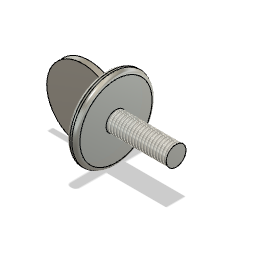
Assembly v1 (Autodesk Fusion 360 archive; units mm, degrees)
design "Pin"
Autodesk Fusion 360 part; units mm, degrees
note: some values were not read from the file. Chosen so that the rebuilt part matches the saved one: a direction; how an offset face is resized.
sketch "Sketch1" plane through (0, 0, 0) normal (1, 0, 0) x (0, 0, -1)
  circle A0 centre (-25, 15) radius 20
  dimension "d1" = 40
  measures "d1" diameter of A0
extrude "Extrude1" add sketch "Sketch1" along normal blind 5
fillet "Fillet1" radius 2 1 edges at (5, 7.7677, 43.6465)
fillet "Fillet2" radius 2 1 edges at (0, 7.7677, 43.6465)
sketch "Sketch2" plane through (5, 0, 0) normal (1, 0, 0) x (0, 0, -1)
  circle A0 centre (-25, 15) radius 18
  circle A1 centre (-25, 15) radius 5
  dimension "d6" = 10
  constraint concentric A0 A1
  measures "d6" diameter of A1
extrude "Extrude2" add sketch "Sketch2" along normal blind 30 contours A1
thread "Thread1" "ISO Metric profile 10.0 M10x1.5 6g" major diameter 9.85 minor diameter 8.141 pitch 1.5 angle 60 resizes the face on face at (25, 14.5022, 20.0248)
sketch "Sketch3" plane through (0, 0, 0) normal (1, 0, 0) x (0, 0, -1)
sketch "Sketch4" plane through (0, 0, 0) normal (-1, 0, 0) x (0, 0, 1)
  circle A0 centre (25, 15) radius 18
sketch "Sketch5" plane through (0, 0, 0) normal (0, 0, 1) x (1, 0, 0)
sketch "Sketch6" plane through (0, 0, 0) normal (0, 0, 1) x (1, 0, 0)
  line L0 (-10, 15) -> (50, 15)
  line L1 (0, 0) -> (0, 29.9666)
  arc A0 (0, 29.9666) -> (0, 0.0334) centre (-10, 15) ccw
  dimension "d9" = 36
  constraint coincident L0.start A0.centre
  constraint coincident L1.start origin
  constraint vertical L1
  constraint coincident L1 A0.end
  measures "d9" diameter of A0
extrude "Extrude3" add sketch "Sketch6" along normal blind 3 from surface at 23.5

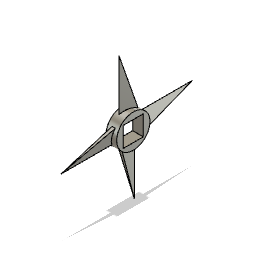
design "Ninja_Star"
Autodesk Fusion 360 part; units mm, degrees
sketch "Sketch1" plane through (0, 0, 0) normal (1, 0, 0) x (0, 0, -1)
  circle A0 centre (0, 0) radius 12.5
  line L0 (7.5, 7.5) -> (-7.5, 7.5)
  line L1 (-7.5, 7.5) -> (-7.5, -7.5)
  line L2 (-7.5, -7.5) -> (7.5, -7.5)
  line L3 (7.5, -7.5) -> (7.5, 7.5)
  line L4 (7.5, 7.5) -> (-7.5, -7.5) construction
  line L5 (-7.5, 7.5) -> (7.5, -7.5) construction
  dimension "d1" = 25
  dimension "d2" = 15
  dimension "d3" = 15
  constraint coincident A0.centre origin
  constraint horizontal L0
  constraint perpendicular L0 L1
  constraint parallel L0 L2
  constraint parallel L1 L3
  constraint coincident L4 A0.centre
  constraint coincident L5 A0.centre
  measures "d1" diameter of A0
  measures "d2" distance of L1.end L2.end
  measures "d3" distance of L0.end L1.end
extrude "Extrude1" add sketch "Sketch1" along normal blind 8
sketch "Sketch2" plane through (0, 0, 0) normal (0, 1, 0) x (1, 0, 0)
sketch "Sketch3" plane through (8, 0, 0) normal (1, 0, 0) x (0, 0, -1)
  line L0 (7.5, 7.5) -> (7.5, -7.5)
  line L1 (7.5, -7.5) -> (-7.5, -7.5)
  line L2 (-7.5, -7.5) -> (-7.5, 7.5)
  line L3 (-7.5, 7.5) -> (7.5, 7.5)
  circle A0 centre (0, 0) radius 12.5
  line L4 (-5.7956, 9.4779) -> (6.4844, 9.4779)
  line L5 (6.4844, 9.4779) -> (-5.7956, 49.4779)
  line L6 (-5.7956, 49.4779) -> (-5.7956, 9.4779)
  dimension "d14" = 40
  constraint perpendicular L0 L4
  constraint perpendicular L4 L6
  measures "d14" distance of L4.start L5.end
extrude "Extrude2" add sketch "Sketch3" along normal blind 2.5 from surface at -5 contours A0 L5 L6
sketch "Sketch4" plane through (0, 0, 0) normal (0, 1, 0) x (1, 0, 0)
  line L0 (2.9867, -5.8624) -> (5.5, -5.8624)
  line L1 (5.5, -5.8624) -> (5.5, 6)
  line L2 (5.5, 6) -> (2.9867, -5.8624)
  constraint horizontal L0
  constraint perpendicular L0 L1
extrude "Extrude3" cut sketch "Sketch4" against normal blind 39 from surface at 50
pattern_circular "C-Pattern1" count 4 over 360 about axis through (1.75, 0, 0) along (1, 0, 0) of "Extrude2", "Extrude3"
sketch "Sketch5" plane through (0, 0, 0) normal (0, 1, 0) x (-1, 0, 0)
sketch "Sketch6" plane through (8, 0, 0) normal (1, 0, 0) x (0, 0, -1)
  line L0 (7.5, 7.5) -> (7.5, -7.5)
  line L1 (7.5, -7.5) -> (-7.5, -7.5)
  line L2 (-7.5, -7.5) -> (-7.5, 7.5)
  line L3 (-7.5, 7.5) -> (7.5, 7.5)
  circle A0 centre (0, 0) radius 12.5
  circle A1 centre (0, 0) radius 12.5
  line L4 (7.5, 7.5) -> (-7.5, 7.5)
  line L5 (-7.5, 7.5) -> (-7.5, -7.5)
  line L6 (-7.5, -7.5) -> (7.5, -7.5)
  line L7 (7.5, -7.5) -> (7.5, 7.5)
  line L8 (7.5, 7.5) -> (-7.5, -7.5) construction
  line L9 (-7.5, 7.5) -> (7.5, -7.5) construction
  constraint coincident A0.centre A1.centre
  constraint horizontal L4
  constraint perpendicular L4 L5
  constraint parallel L4 L6
  constraint parallel L5 L7
  constraint coincident L0.start L3.end
  constraint coincident L8 A0.centre
  constraint coincident L9 A0.centre
extrude "Extrude4" add sketch "Sketch6" against normal blind 8

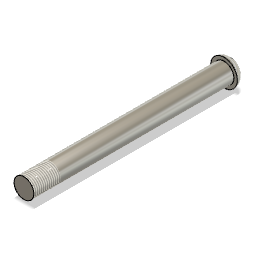
design "HandlePin"
Autodesk Fusion 360 part; units mm, degrees
sketch "Sketch1" plane through (0, 0, 0) normal (0, 0, 1) x (1, 0, 0)
  circle A0 centre (74.2368, 105.6989) radius 7.5
  dimension "d13" = 15
  measures "d13" diameter of A0
extrude "Extrude1" add sketch "Sketch1" along normal blind 150
sketch "Sketch2" plane through (0, 0, 0) normal (0, 0, -1) x (-1, 0, 0)
  circle A0 centre (-74.2368, 105.6989) radius 7.5
  circle A1 centre (-74.2368, 105.6989) radius 10
  dimension "d16" = 20
  constraint horizontal A0.centre A1.centre
  constraint concentric A0 A1
  measures "d16" diameter of A1
extrude "Extrude2" add sketch "Sketch2" along normal blind 6 draft 6 contours A0 | A1
fillet "Fillet1" radius 6 1 edges at (84.148, 109.5431, -6)
sketch "Sketch3" plane through (0, 0, -6) normal (0, 0, -1) x (-1, 0, 0)
  circle A0 centre (-74.2368, 105.6989) radius 4
  line L0 (-75.2368, 112.1989) -> (-73.2368, 112.1989)
  line L1 (-73.2368, 112.1989) -> (-73.2368, 99.1989)
  line L2 (-73.2368, 99.1989) -> (-75.2368, 99.1989)
  line L3 (-75.2368, 99.1989) -> (-75.2368, 112.1989)
  dimension "d20" = 2
  dimension "d21" = 1
  dimension "d22" = 6.5
  constraint horizontal L0
  constraint vertical L1
  constraint horizontal L2
  constraint vertical L3
  measures "d20" distance of L0.start L0.end
  measures "d21" distance of A0.centre L1
  measures "d22" distance of A0.centre L2
extrude "Extrude3" cut sketch "Sketch3" against normal blind 2 contours A0 L1 L3 | A0 L0 L1 L3 | A0 L1 L2 L3
thread "Thread1" "ISO Metric profile 15.0 M15x1.5 6g" major diameter 14.85 minor diameter 13.1369 pitch 1.5 angle 60 resizes the face on face at (81.7275, 105.325, 100)

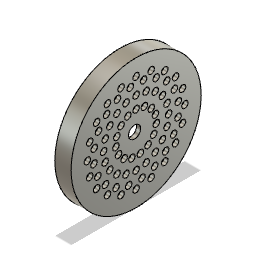
design "SHAPER"
Autodesk Fusion 360 part; units mm, degrees
sketch "Sketch1" plane through (0, 0, 0) normal (1, 0, 0) x (0, 0, -1)
  circle A0 centre (0, 0) radius 80
  circle A1 centre (0, 0) radius 70
  dimension "d1" = 160
  dimension "d2" = 140
  constraint coincident A0.centre A1.centre
  measures "d1" diameter of A0
  measures "d2" diameter of A1
extrude "Extrude1" add sketch "Sketch1" along normal blind 15
thread "Thread1" "ISO Metric profile 140.0 M140x8 6H" major diameter 140.8024 minor diameter 131.8397 pitch 8 angle 60 resizes the face on face at (10, -6.9697, -69.6522)
sketch "Sketch2" plane through (15, 0, 0) normal (1, 0, 0) x (0, 0, -1)
  circle A0 centre (0, 0) radius 65.9198
  circle A1 centre (0, 0) radius 80
  circle A2 centre (0, 0) radius 80
  constraint concentric A0 A2
extrude "Extrude2" add sketch "Sketch2" along normal blind 5 contours A0 | A1 A2
hole "Hole1" at (20, 1.6801, 1.9117) direction (-1, 0, 0) diameter 15 depth 40 tip angle 180
sketch "Sketch3" plane through (20, 0, 0) normal (1, 0, 0) x (0, 0, -1)
  circle A0 centre (-1.9117, 1.6801) radius 7.5
  circle A1 centre (0, 0) radius 80
  point P0 (0, 60)
hole "Hole2" at (20, 60, 0) direction (-1, 0, 0) diameter 8 depth 40 tip angle 180
pattern_circular "C-Pattern1" count 20 over 360 about axis through (1.75, 0, 0) along (1, 0, 0) of "Hole2"
sketch "Sketch4" plane through (20, 0, 0) normal (1, 0, 0) x (0, 0, -1)
  circle A0 centre (18.541, 57.0634) radius 4
  circle A1 centre (35.2671, 48.541) radius 4
  circle A2 centre (48.541, 35.2671) radius 4
  circle A3 centre (57.0634, 18.541) radius 4
  circle A4 centre (60, 0) radius 4
  circle A5 centre (57.0634, -18.541) radius 4
  circle A6 centre (48.541, -35.2671) radius 4
  circle A7 centre (35.2671, -48.541) radius 4
  circle A8 centre (18.541, -57.0634) radius 4
  circle A9 centre (0, -60) radius 4
  circle A10 centre (-18.541, -57.0634) radius 4
  circle A11 centre (-35.2671, -48.541) radius 4
  circle A12 centre (-48.541, -35.2671) radius 4
  circle A13 centre (-57.0634, -18.541) radius 4
  circle A14 centre (-60, 0) radius 4
  circle A15 centre (-57.0634, 18.541) radius 4
  circle A16 centre (-48.541, 35.2671) radius 4
  circle A17 centre (-35.2671, 48.541) radius 4
  circle A18 centre (-18.541, 57.0634) radius 4
  circle A19 centre (0, 60) radius 4
  circle A20 centre (-1.9117, 1.6801) radius 7.5
  circle A21 centre (0, 0) radius 80
  point P0 (-7.2239, 51.8768)
hole "Hole3" at (20, 51.8768, 7.2239) direction (-1, 0, 0) diameter 8 depth 40 tip angle 180
pattern_circular "C-Pattern2" count 20 over 360 about axis through (1.75, 0, 0) along (1, 0, 0) of "Hole3"
sketch "Sketch5" plane through (20, 0, 0) normal (1, 0, 0) x (0, 0, -1)
  circle A0 centre (9.1605, 51.5701) radius 4
  circle A1 centre (24.6482, 46.2153) radius 4
  circle A2 centre (37.7231, 36.3367) radius 4
  circle A3 centre (47.1055, 22.9012) radius 4
  circle A4 centre (51.8768, 7.2239) radius 4
  circle A5 centre (51.5701, -9.1605) radius 4
  circle A6 centre (46.2153, -24.6482) radius 4
  circle A7 centre (36.3367, -37.7231) radius 4
  circle A8 centre (22.9012, -47.1055) radius 4
  circle A9 centre (7.2239, -51.8768) radius 4
  circle A10 centre (-9.1605, -51.5701) radius 4
  circle A11 centre (-24.6482, -46.2153) radius 4
  circle A12 centre (-37.7231, -36.3367) radius 4
  circle A13 centre (-47.1055, -22.9012) radius 4
  circle A14 centre (-51.8768, -7.2239) radius 4
  circle A15 centre (-51.5701, 9.1605) radius 4
  circle A16 centre (-46.2153, 24.6482) radius 4
  circle A17 centre (-36.3367, 37.7231) radius 4
  circle A18 centre (-22.9012, 47.1055) radius 4
  circle A19 centre (-7.2239, 51.8768) radius 4
  circle A20 centre (18.541, 57.0634) radius 4
  circle A21 centre (35.2671, 48.541) radius 4
  circle A22 centre (48.541, 35.2671) radius 4
  circle A23 centre (57.0634, 18.541) radius 4
  circle A24 centre (60, 0) radius 4
  circle A25 centre (57.0634, -18.541) radius 4
  circle A26 centre (48.541, -35.2671) radius 4
  circle A27 centre (35.2671, -48.541) radius 4
  circle A28 centre (18.541, -57.0634) radius 4
  circle A29 centre (0, -60) radius 4
  circle A30 centre (-18.541, -57.0634) radius 4
  circle A31 centre (-35.2671, -48.541) radius 4
  circle A32 centre (-48.541, -35.2671) radius 4
  circle A33 centre (-57.0634, -18.541) radius 4
  circle A34 centre (-60, 0) radius 4
  circle A35 centre (-57.0634, 18.541) radius 4
  circle A36 centre (-48.541, 35.2671) radius 4
  circle A37 centre (-35.2671, 48.541) radius 4
  circle A38 centre (-18.541, 57.0634) radius 4
  circle A39 centre (0, 60) radius 4
  circle A40 centre (-1.9117, 1.6801) radius 7.5
  circle A41 centre (0, 0) radius 80
  point P0 (0, 40)
hole "Hole4" at (20, 40, 0) direction (-1, 0, 0) diameter 8 depth 40 tip angle 180
pattern_circular "C-Pattern3" count 20 over 360 about axis through (1.75, 0, 0) along (1, 0, 0) of "Hole4"
sketch "Sketch6" plane through (20, 0, 0) normal (1, 0, 0) x (0, 0, -1)
  circle A0 centre (12.3607, 38.0423) radius 4
  circle A1 centre (23.5114, 32.3607) radius 4
  circle A2 centre (32.3607, 23.5114) radius 4
  circle A3 centre (38.0423, 12.3607) radius 4
  circle A4 centre (40, 0) radius 4
  circle A5 centre (38.0423, -12.3607) radius 4
  circle A6 centre (32.3607, -23.5114) radius 4
  circle A7 centre (23.5114, -32.3607) radius 4
  circle A8 centre (12.3607, -38.0423) radius 4
  circle A9 centre (0, -40) radius 4
  circle A10 centre (-12.3607, -38.0423) radius 4
  circle A11 centre (-23.5114, -32.3607) radius 4
  circle A12 centre (-32.3607, -23.5114) radius 4
  circle A13 centre (-38.0423, -12.3607) radius 4
  circle A14 centre (-40, 0) radius 4
  circle A15 centre (-38.0423, 12.3607) radius 4
  circle A16 centre (-32.3607, 23.5114) radius 4
  circle A17 centre (-23.5114, 32.3607) radius 4
  circle A18 centre (-12.3607, 38.0423) radius 4
  circle A19 centre (0, 40) radius 4
  circle A20 centre (9.1605, 51.5701) radius 4
  circle A21 centre (24.6482, 46.2153) radius 4
  circle A22 centre (37.7231, 36.3367) radius 4
  circle A23 centre (47.1055, 22.9012) radius 4
  circle A24 centre (51.8768, 7.2239) radius 4
  circle A25 centre (51.5701, -9.1605) radius 4
  circle A26 centre (46.2153, -24.6482) radius 4
  circle A27 centre (36.3367, -37.7231) radius 4
  circle A28 centre (22.9012, -47.1055) radius 4
  circle A29 centre (7.2239, -51.8768) radius 4
  circle A30 centre (-9.1605, -51.5701) radius 4
  circle A31 centre (-24.6482, -46.2153) radius 4
  circle A32 centre (-37.7231, -36.3367) radius 4
  circle A33 centre (-47.1055, -22.9012) radius 4
  circle A34 centre (-51.8768, -7.2239) radius 4
  circle A35 centre (-51.5701, 9.1605) radius 4
  circle A36 centre (-46.2153, 24.6482) radius 4
  circle A37 centre (-36.3367, 37.7231) radius 4
  circle A38 centre (-22.9012, 47.1055) radius 4
  circle A39 centre (-7.2239, 51.8768) radius 4
  circle A40 centre (18.541, 57.0634) radius 4
  circle A41 centre (35.2671, 48.541) radius 4
  circle A42 centre (48.541, 35.2671) radius 4
  circle A43 centre (57.0634, 18.541) radius 4
  circle A44 centre (60, 0) radius 4
  circle A45 centre (57.0634, -18.541) radius 4
  circle A46 centre (48.541, -35.2671) radius 4
  circle A47 centre (35.2671, -48.541) radius 4
  circle A48 centre (18.541, -57.0634) radius 4
  circle A49 centre (0, -60) radius 4
  circle A50 centre (-18.541, -57.0634) radius 4
  circle A51 centre (-35.2671, -48.541) radius 4
  circle A52 centre (-48.541, -35.2671) radius 4
  circle A53 centre (-57.0634, -18.541) radius 4
  circle A54 centre (-60, 0) radius 4
  circle A55 centre (-57.0634, 18.541) radius 4
  circle A56 centre (-48.541, 35.2671) radius 4
  circle A57 centre (-35.2671, 48.541) radius 4
  circle A58 centre (-18.541, 57.0634) radius 4
  circle A59 centre (0, 60) radius 4
  circle A60 centre (-1.9117, 1.6801) radius 7.5
  circle A61 centre (0, 0) radius 80
  point P0 (0, 25)
hole "Hole5" at (20, 25, 0) direction (-1, 0, 0) diameter 8 depth 40 tip angle 180
pattern_circular "C-Pattern4" count 15 over 360 about axis through (1.75, 0, 0) along (1, 0, 0) of "Hole5"

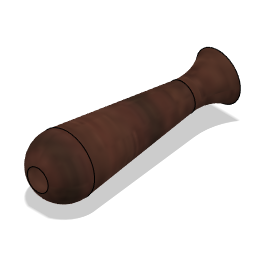
design "Handle v0"
Autodesk Fusion 360 part; units mm, degrees
sketch "Sketch1" plane through (0, 0, 0) normal (1, 0, 0) x (0, 0, -1)
  line L0 (-0.8619, 0) -> (130, 0)
  line L1 (130, 0) -> (130, 15.8604)
  line L2 (104.0572, 9.4893) -> (21.572, 19.8034)
  arc A0 (104.0572, 9.4893) -> (130, 15.8604) centre (108.6974, 46.5989) ccw
  arc A1 (21.572, 19.8034) -> (-0.8619, 0) centre (19.0957, 0) ccw
  constraint horizontal L0
  constraint perpendicular L0 L1
  constraint coincident L0 A1.centre
  constraint tangent L2 A1
  constraint tangent L2 A0
revolve "Revolve1" add sketch "Sketch1" angle 360 about axis through (0, 0, 1.75) along (0, 0, 1) makes body 1
sketch "Sketch2" plane through (0, 0, -130) normal (0, 0, -1) x (-1, 0, 0)
  circle A0 centre (0, 0) radius 15.8604
  circle A1 centre (0, 0) radius 7.5
  circle A2 centre (0, 0) radius 19.8034
  dimension "d2" = 15
  constraint concentric A1 A2
  measures "d2" diameter of A1
extrude "Extrude1" cut sketch "Sketch2" against normal through all contours A1 bodies 1
copy_body "Body->Comp1" bodies 1 removing the originals makes body 2 in component "Component"
component "Component" placed x (1, 0, 0) y (0, 1, 0) z (0, 0, 1) at (0, 0, 0)
